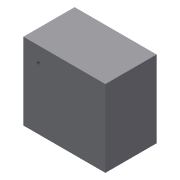
# Autodesk Inventor part: ChamberV4
Saved by Autodesk Inventor 2013 (Build 170138000, 138)
## iProperties
Created: 2014-11-20
Part Number: ChamberV4
Material: Generic
Document SubType Name: Modeling
Designer: 120pa
Density: 1 g/cm^3
Author: 120pa
Autodesk Inventor part; units mm, degrees
ref_plane "YZ Plane" through (0, 0, 0) normal (1, 0, 0) x (0, 1, 0)
ref_plane "XZ Plane" through (0, 0, 0) normal (0, 1, 0) x (-1, 0, 0)
ref_plane "XY Plane" through (0, 0, 0) normal (0, 0, 1) x (1, 0, 0)
sketch "Sketch1" plane through (0, 0, 0) normal (0, 1, 0) x (-1, 0, 0)
  line L0 (-14.0227, -4.1785) -> (45.9773, -4.1785)
  line L1 (45.9773, -4.1785) -> (45.9773, 55.8215)
  line L2 (45.9773, 55.8215) -> (-14.0227, 55.8215)
  line L3 (-14.0227, 55.8215) -> (-14.0227, -4.1785)
  point P0 (0, 0)
  dimension "d4" = 60
  dimension "d7" = 60
  constraints: 8 end point, 3 perpendicular
  measures "d4" distance of L1.end L2.end
  measures "d7" distance of L2.end L0.start
extrude "Extrusion1" add sketch "Sketch1" along normal blind 50
sketch "Sketch2" plane through (0, 50, 0) normal (0, 1, 0) x (1, 0, 0)
  line L0 (-30.9773, -10.8215) -> (11.0227, -10.8215)
  line L1 (11.0227, -10.8215) -> (11.0227, -50.8215)
  line L2 (11.0227, -50.8215) -> (-30.9773, -50.8215)
  line L3 (-30.9773, -50.8215) -> (-30.9773, -10.8215)
  line L4 (14.0227, 4.1785) -> (-45.9773, 4.1785) projected
  line L5 (-45.9773, 4.1785) -> (-45.9773, -55.8215) projected
  line L6 (-45.9773, -55.8215) -> (14.0227, -55.8215) projected
  line L7 (14.0227, -55.8215) -> (14.0227, 4.1785) projected
  point P0 (0, 0)
  dimension "d8" = 15
  dimension "d9" = 15
  dimension "d10" = 3
  dimension "d11" = 5
  constraints: 8 end point
  measures "d8" distance between parallel lines of L4 L0
  measures "d9" distance between parallel lines of L5 L3
  measures "d10" distance between parallel lines of L7 L1
  measures "d11" distance between parallel lines of L2 L6
extrude "Extrusion2" cut sketch "Sketch2" against normal blind 46 contours L0 L1 L2 L3
sketch "Sketch3" plane through (14.0227, 0, -4.1785) normal (0, 0, -1) x (-1, 0, 0)
  line L0 (60, 0) -> (60, 50) projected
  line L1 (0, 50) -> (60, 50) projected
  circle A0 centre (30, 25) radius 21
  point P0 (14.0227, 0)
  dimension "d12" = 25
  dimension "d13" = 30
  dimension "d14" = 42
  constraints: 1 centre point
  measures "d12" distance from line of L1 A0.centre
  measures "d13" distance from line of L0 A0.centre
  measures "d14" diameter of A0
extrude "Extrusion3" cut sketch "Sketch3" against normal blind 30
sketch "Sketch4" plane through (-45.9773, 0, -4.1785) normal (-1, 0, 0) x (0, 0, 1)
  line L0 (0, 50) -> (60, 50) projected
  line L1 (0, 0) -> (0, 50) projected
  circle A0 centre (30, 25) radius 16
  point P0 (4.1785, 0)
  dimension "d17" = 25
  dimension "d18" = 30
  dimension "d19" = 32
  constraints: 1 centre point
  measures "d17" distance from line of L0 A0.centre
  measures "d18" distance from line of L1 A0.centre
  measures "d19" diameter of A0
extrude "Extrusion4" cut sketch "Sketch4" against normal blind 30
sketch "Sketch5" plane through (14.0227, 0, -4.1785) normal (0, 0, -1) x (-1, 0, 0)
  point P0 (14.0227, 0)
extrude "Extrusion5" [suppressed]
fillet "Fillet7" radius 20 1 edges at (-30.9773, 27, 50.8215)
fillet "Fillet8" radius 2 2 edges at (11.0227, 27, 50.8215) (11.0227, 27, 10.8215)
sketch "Sketch10" plane through (0, 50, 0) normal (0, 1, 0) x (1, 0, 0)
  line L0 (-45.9773, 4.1785) -> (-45.9773, -55.8215) projected
  line L1 (-45.9773, -55.8215) -> (14.0227, -55.8215) projected
  circle A0 centre (-33.9773, -48.8215) radius 1.7819
  point P0 (0, 0)
  dimension "d71" = 7
  dimension "d72" = 12
  constraints: 1 centre point
  measures "d71" distance from line of L1 A0.centre
  measures "d72" distance from line of L0 A0.centre
hole "Hole1" at (-33.9773, 50, 48.8215) direction (0, -1, 0) diameter 6.4 depth 30 tip angle 118
fillet "Fillet9" radius 10 2 edges at (-30.9773, 44.8485, 10.8215) (-30.9773, 7.1515, 10.8215)
sketch "Sketch15" plane through (14.0227, 0, -4.1785) normal (0, 0, -1) x (-1, 0, 0)
  circle A0 centre (30, 25) radius 21 projected
  line L0 (0, 0) -> (60, 0) projected
  line L1 (60, 0) -> (60, 50) projected
  line L2 (0, 50) -> (60, 50) projected
  line L3 (0, 0) -> (0, 50) projected
  point P0 (14.0227, 0)
extrude "Extrusion12" add sketch "Sketch15" along normal blind 15
sketch "Sketch16" plane through (14.0227, 0, -19.1785) normal (0, 0, -1) x (-1, 0, 0)
  line L0 (48, 7) -> (12, 7)
  line L1 (12, 7) -> (12, 43)
  line L2 (12, 43) -> (48, 43)
  line L3 (48, 43) -> (48, 7)
  line L4 (48, 7) -> (12, 43) construction
  line L5 (12, 7) -> (48, 43) construction
  point P0 (14.0227, 0)
  point P1 (30, 25)
  dimension "d105" = 36
  dimension "d106" = 36
  constraints: 12 end point, 2 midpoint
  measures "d105" distance of L1.end L2.end
  measures "d106" distance of L0.end L1.end
hole "Hole4" at (2.0227, 43, -19.1785) at (-33.9773, 43, -19.1785) at (-33.9773, 7, -19.1785) at (2.0227, 7, -19.1785) direction (0, 0, 1) diameter 2.156 depth 8 tip angle 118 thread size "4-40 UNC" class "2B" standard "ANSI Unified Screw Threads"
sketch "Sketch17" plane through (-45.9773, 0, 55.8215) normal (-1, 0, 0) x (0, 0, 1)
  circle A0 centre (-30, 25) radius 16 projected
  line L0 (0, 0) -> (-75, 0) projected
  line L1 (0, 0) -> (0, 50) projected
  line L2 (0, 50) -> (-75, 50) projected
  line L3 (-75, 0) -> (-75, 50) projected
  point P0 (-55.8215, 0)
extrude "Extrusion13" add sketch "Sketch17" along normal blind 20
sketch "Sketch18" plane through (-65.9773, 0, 55.8215) normal (-1, 0, 0) x (0, 0, 1)
  line L0 (-15, 10) -> (-45, 10)
  line L1 (-45, 10) -> (-45, 40)
  line L2 (-45, 40) -> (-15, 40)
  line L3 (-15, 40) -> (-15, 10)
  line L4 (-15, 10) -> (-45, 40) construction
  line L5 (-45, 10) -> (-15, 40) construction
  point P0 (-55.8215, 0)
  point P1 (-30, 25)
  dimension "d116" = 30
  dimension "d117" = 30
  constraints: 12 end point, 2 midpoint
  measures "d116" distance of L1.end L2.end
  measures "d117" distance of L0.end L1.end
hole "Hole5" at (-65.9773, 40, 10.8215) at (-65.9773, 40, 40.8215) at (-65.9773, 10, 40.8215) at (-65.9773, 10, 10.8215) direction (1, 0, 0) diameter 2.156 depth 8 tip angle 118 thread size "4-40 UNC" class "2B" standard "ANSI Unified Screw Threads"
hole "Hole6" at (-50.9773, 0, 40.8215) direction (0, 1, 0) diameter 3.302 depth 8 tip angle 118 thread size "8-32 UNC" class "2B" standard "ANSI Unified Screw Threads"
body "Solid1"
